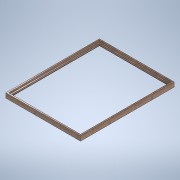
# Autodesk Inventor part: solar panels holder
Saved by Autodesk Inventor 2020 (Build 240168000, 168)
## iProperties
Created: 2020-06-26
Part Number: solar panels holder
Material: Generic
Document SubType Name: Modeling
Designer: Abbas
Density: 1 g/cm^3
Appearance: Default
Author: Abbas
Autodesk Inventor part; units mm, degrees
ref_plane "YZ Plane" through (0, 0, 0) normal (1, 0, 0) x (0, 1, 0)
ref_plane "XZ Plane" through (0, 0, 0) normal (0, 1, 0) x (-1, 0, 0)
ref_plane "XY Plane" through (0, 0, 0) normal (0, 0, 1) x (1, 0, 0)
sketch "Sketch1" plane through (0, 0, 0) normal (0, 1, 0) x (-1, 0, 0)
  line L0 (533, 674) -> (-533, 674)
  line L1 (-533, 674) -> (-533, -674)
  line L2 (-533, -674) -> (533, -674)
  line L3 (533, -674) -> (533, 674)
  line L4 (533, 674) -> (-533, -674) construction
  line L5 (-533, 674) -> (533, -674) construction
  line L6 (553, 694) -> (-553, 694)
  line L7 (-553, 694) -> (-553, -694)
  line L8 (-553, -694) -> (553, -694)
  line L9 (553, -694) -> (553, 694)
  line L10 (553, 694) -> (-553, -694) construction
  line L11 (-553, 694) -> (553, -694) construction
  line L12 (513, 654) -> (-513, 654)
  line L13 (-513, 654) -> (-513, -654)
  line L14 (-513, -654) -> (513, -654)
  line L15 (513, -654) -> (513, 654)
  line L16 (513, 654) -> (-513, -654) construction
  line L17 (-513, 654) -> (513, -654) construction
  point P0 (0, 0)
  dimension "d0" = 1066
  dimension "d1" = 1348
  dimension "d2" = 1106
  dimension "d3" = 1388
  dimension "d4" = 1026
  dimension "d5" = 1308
  constraints: 36 end point, 6 midpoint, 6 parallel, 3 horizontal, 3 perpendicular
  measures "d0" distance of L2.end L1.end
  measures "d1" distance of L1.end L0.end
  measures "d2" distance of L8.end L7.end
  measures "d3" distance of L7.end L6.end
  measures "d4" distance of L14.end L13.end
  measures "d5" distance of L13.end L12.end
extrude "Extrusion2" add sketch "Sketch1" along normal mid plane 20 contours L3 L2 L1 L0
extrude "Extrusion3" add sketch "Sketch1" along normal mid plane 70 contours L9 L8 L7 L6
body "Solid2"
